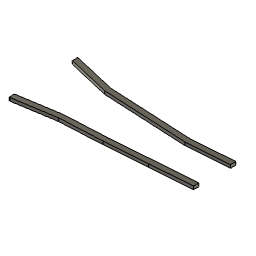
ArmTopView v2 (Autodesk Fusion 360 design; units mm, degrees)
Autodesk Fusion 360 part; units mm, degrees
sketch "Sketch1" plane through (0, 0, 0) normal (0, 0, 1) x (1, 0, 0)
  line L0 (-23.4246, -53.2136) -> (16.5754, -62.6036)
  line L1 (16.5754, -62.6036) -> (56.5754, -64.6036)
  line L2 (56.5754, -64.6036) -> (96.5754, -66.6036)
  line L3 (96.5754, -66.6036) -> (136.5754, -63.6036)
  line L4 (-23.4246, -107.9936) -> (16.5754, -101.6036)
  line L5 (16.5754, -101.6036) -> (56.5754, -99.6036)
  line L6 (56.5754, -99.6036) -> (96.5754, -96.6036)
  line L7 (96.5754, -96.6036) -> (136.5754, -93.6036)
  line L8 (-22.2819, -48.3459) -> (17.2773, -57.6324)
  line L9 (17.2773, -57.6324) -> (56.8251, -59.6098)
  line L10 (56.8251, -59.6098) -> (96.5131, -61.5942)
  line L11 (96.5131, -61.5942) -> (136.2015, -58.6176)
  line L12 (-22.6358, -112.931) -> (17.0962, -106.5838)
  line L13 (17.0962, -106.5838) -> (56.8873, -104.5942)
  line L14 (56.8873, -104.5942) -> (96.9494, -101.5896)
  line L15 (-23.4246, -53.2136) -> (-23.4246, -48.2136)
  line L16 (-23.4246, -107.9936) -> (-23.4246, -112.9936)
  line L17 (136.5754, -93.6036) -> (136.5754, -98.6036)
  line L18 (136.5754, -63.6036) -> (136.5754, -58.6036)
  line L19 (-23.4246, -48.2136) -> (-22.2819, -48.3459)
  line L20 (-23.4246, -112.9936) -> (-22.6358, -112.931)
  line L21 (96.9494, -101.5896) -> (136.5754, -98.6036)
  line L22 (136.2015, -58.6176) -> (136.5754, -58.6036)
  dimension "d1" = 54.78
  dimension "d21" = -5
  dimension "d23" = 5
  dimension "d24" = 5
  dimension "d25" = 5
  dimension "d26" = 5
  constraint parallel L6 L7
  constraint vertical L15
  constraint vertical L16
  constraint vertical L17
  constraint vertical L18
  measures "d1" distance of L4.start L0.start
  measures "d23" distance of L0.start L15.end
  measures "d24" distance of L3.end L18.end
  measures "d25" distance of L7.end L17.end
  measures "d26" distance of L4.start L16.end
extrude "Extrude1" add sketch "Sketch1" along normal blind 3 makes body 1 at (96.7001, -98.2656, 0) makes body 2 at (43.4761, -62.2799, 0)
